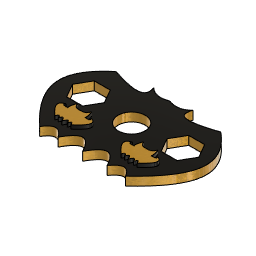
batman_fidget_spinner_darshan_nair (Autodesk Fusion 360 design; units mm, degrees)
Autodesk Fusion 360 part; units mm, degrees
sketch "Sketch1" plane through (0, 0, 0) normal (0, 0, 1) x (1, 0, 0)
  line L0 (0, 0) -> (0, 11)
  spline S0 degree 5 poles (0, 31) (0.3798, 30.869) (1.1341, 30.6235) (2.2502, 30.3047) (3.7068, 29.9801) (5.4716, 29.7535) (7.1751, 29.7226) (8.812, 29.9045) (10.3789, 30.3103) (11.8777, 30.9337) (13.3133, 31.7593) (14.4152, 32.5687) (15.217, 33.2543) (15.7408, 33.7457) (16, 34) knots 0 0 0 0 0 0 0.1 0.2 0.3 0.4 0.5 0.6 0.7 0.8 0.9 1 1 1 1 1 1
  spline S1 degree 5 poles (16, 34) (15.7635, 33.3498) (15.3667, 32.1059) (15.0006, 30.4093) (14.9782, 28.4915) (15.7664, 26.6977) (17.4106, 25.5367) (19.9066, 25.0054) (23.1867, 25.0538) (27.1658, 25.6189) (31.7601, 26.6389) (35.8754, 27.78) (39.1911, 28.8054) (41.5017, 29.563) (42.6821, 29.9604) knots 0 0 0 0 0 0 0.1 0.2 0.3 0.4 0.5 0.6 0.7 0.8 0.9 1 1 1 1 1 1
  spline S2 degree 5 poles (42.6821, 29.9604) (44.1584, 28.7477) (46.9634, 26.3054) (50.7286, 22.5913) (54.8497, 17.5364) (58.4053, 11.0351) (60.241, 4.3371) (60.2452, -2.5706) (58.4098, -9.6887) (54.8568, -17.0034) (49.7384, -24.4973) (44.5047, -30.6226) (39.9812, -35.2851) (36.704, -38.4234) (35, -40) knots 0 0 0 0 0 0 0.1 0.2 0.3 0.4 0.5 0.6 0.7 0.8 0.9 1 1 1 1 1 1
  spline S3 degree 5 poles (35, -40) (34.7252, -39.5521) (34.1734, -38.6959) (33.3391, -37.5297) (32.2132, -36.2152) (30.7816, -34.9998) (29.3239, -34.2492) (27.8379, -33.9997) (26.3228, -34.2679) (24.7799, -35.0299) (23.2114, -36.247) (21.9378, -37.5541) (20.9727, -38.7099) (20.3249, -39.5572) (20, -40) knots 0 0 0 0 0 0 0.1 0.2 0.3 0.4 0.5 0.6 0.7 0.8 0.9 1 1 1 1 1 1
  spline S4 degree 5 poles (20, -40) (19.6, -39.2415) (18.8, -37.7908) (17.6, -35.8134) (16, -33.581) (14, -31.5094) (12, -30.2211) (10, -29.7801) (8, -30.2211) (6, -31.5094) (4, -33.581) (2.4, -35.8134) (1.2, -37.7908) (0.4, -39.2415) (0, -40) knots 0 0 0 0 0 0 0.1 0.2 0.3 0.4 0.5 0.6 0.7 0.8 0.9 1 1 1 1 1 1
  spline S5 degree 5 poles (0, 31) (-0.3798, 30.869) (-1.1341, 30.6235) (-2.2502, 30.3047) (-3.7068, 29.9801) (-5.4716, 29.7535) (-7.1751, 29.7226) (-8.812, 29.9045) (-10.3789, 30.3103) (-11.8777, 30.9337) (-13.3133, 31.7593) (-14.4152, 32.5687) (-15.217, 33.2543) (-15.7408, 33.7457) (-16, 34) knots 0 0 0 0 0 0 0.1 0.2 0.3 0.4 0.5 0.6 0.7 0.8 0.9 1 1 1 1 1 1
  line L1 (-1.8866, 31.6508) -> (1.8866, 30.3492)
  line L2 (14.6318, 32.6578) -> (17.3682, 35.3422)
  line L3 (1.8866, 31.6508) -> (-1.8866, 30.3492)
  line L4 (-14.6318, 32.6578) -> (-17.3682, 35.3422)
  spline S6 degree 5 poles (-16, 34) (-15.7635, 33.3498) (-15.3667, 32.1059) (-15.0006, 30.4093) (-14.9782, 28.4915) (-15.7664, 26.6977) (-17.4106, 25.5367) (-19.9066, 25.0054) (-23.1867, 25.0538) (-27.1658, 25.6189) (-31.7601, 26.6389) (-35.8754, 27.78) (-39.1911, 28.8054) (-41.5017, 29.563) (-42.6821, 29.9604) knots 0 0 0 0 0 0 0.1 0.2 0.3 0.4 0.5 0.6 0.7 0.8 0.9 1 1 1 1 1 1
  line L5 (17.5567, 38.2791) -> (14.4433, 29.7209)
  line L6 (38.3421, 28.4994) -> (47.0222, 31.4213)
  line L7 (-17.5567, 38.2791) -> (-14.4433, 29.7209)
  line L8 (-38.3421, 28.4994) -> (-47.0222, 31.4213)
  spline S7 degree 5 poles (-42.6821, 29.9604) (-44.1584, 28.7477) (-46.9634, 26.3054) (-50.7286, 22.5913) (-54.8497, 17.5364) (-58.4053, 11.0351) (-60.241, 4.3371) (-60.2452, -2.5706) (-58.4098, -9.6887) (-54.8568, -17.0034) (-49.7384, -24.4973) (-44.5047, -30.6226) (-39.9812, -35.2851) (-36.704, -38.4234) (-35, -40) knots 0 0 0 0 0 0 0.1 0.2 0.3 0.4 0.5 0.6 0.7 0.8 0.9 1 1 1 1 1 1
  line L9 (34.9577, 36.3058) -> (50.4066, 23.6149)
  line L10 (42.7125, -32.864) -> (27.2875, -47.136)
  line L11 (-34.9577, 36.3058) -> (-50.4066, 23.6149)
  line L12 (-42.7125, -32.864) -> (-27.2875, -47.136)
  spline S8 degree 5 poles (-35, -40) (-34.7252, -39.5521) (-34.1734, -38.6959) (-33.3391, -37.5297) (-32.2132, -36.2152) (-30.7816, -34.9998) (-29.3239, -34.2492) (-27.8379, -33.9997) (-26.3228, -34.2679) (-24.7799, -35.0299) (-23.2114, -36.247) (-21.9378, -37.5541) (-20.9727, -38.7099) (-20.3249, -39.5572) (-20, -40) knots 0 0 0 0 0 0 0.1 0.2 0.3 0.4 0.5 0.6 0.7 0.8 0.9 1 1 1 1 1 1
  line L13 (36.1955, -41.9484) -> (33.8045, -38.0516)
  line L14 (21.3607, -38.1457) -> (18.6393, -41.8543)
  line L15 (-36.1955, -41.9484) -> (-33.8045, -38.0516)
  line L16 (-21.3607, -38.1457) -> (-18.6393, -41.8543)
  spline S9 degree 5 poles (-20, -40) (-19.6, -39.2415) (-18.8, -37.7908) (-17.6, -35.8134) (-16, -33.581) (-14, -31.5094) (-12, -30.2211) (-10, -29.7801) (-8, -30.2211) (-6, -31.5094) (-4, -33.581) (-2.4, -35.8134) (-1.2, -37.7908) (-0.4, -39.2415) (0, -40) knots 0 0 0 0 0 0 0.1 0.2 0.3 0.4 0.5 0.6 0.7 0.8 0.9 1 1 1 1 1 1
  line L17 (21.5767, -42.9909) -> (18.4233, -37.0091)
  line L18 (1.5794, -37.0105) -> (-1.5794, -42.9895)
  line L19 (-21.5767, -42.9909) -> (-18.4233, -37.0091)
  line L20 (-1.5794, -37.0105) -> (1.5794, -42.9895)
  circle A0 centre (0, 0) radius 11.05
  spline S10 degree 5 poles (-27, -15) (-26.7311, -15.0239) (-26.2109, -15.056) (-25.4835, -15.0575) (-24.6198, -14.9657) (-23.7179, -14.6962) (-22.9921, -14.2817) (-22.4353, -13.7442) (-22.0319, -13.1243) (-21.7558, -12.4856) (-21.5648, -11.9235) (-21.41, -11.5448) (-21.2469, -11.4404) (-21.0459, -11.6596) (-20.8038, -12.1839) (-20.5351, -12.9481) (-20.2662, -13.8594) (-20.0277, -14.8166) (-19.8481, -15.7276) (-19.7461, -16.5309) (-19.7315, -17.1925) (-19.793, -17.5959) (-19.8805, -17.826) (-19.9571, -17.9474) (-20, -18) knots 0 0 0 0 0 0 0.05 0.1 0.15 0.2 0.25 0.3 0.35 0.4 0.45 0.5 0.55 0.6 0.65 0.7 0.75 0.8 0.85 0.9 0.95 1 1 1 1 1 1
  spline S11 degree 5 poles (-20, -18) (-19.8028, -18.0252) (-19.4192, -18.0705) (-18.8763, -18.1231) (-18.2187, -18.1622) (-17.5153, -18.1555) (-16.9428, -18.0872) (-16.5158, -17.9507) (-16.247, -17.7399) (-16.1405, -17.4529) (-16.1886, -17.0932) (-16.3429, -16.7512) (-16.5199, -16.4659) (-16.6648, -16.263) (-16.7439, -16.1585) knots 0 0 0 0 0 0 0.1 0.2 0.3 0.4 0.5 0.6 0.7 0.8 0.9 1 1 1 1 1 1
  spline S12 degree 5 poles (-16.7439, -16.1585) (-16.3983, -16.2667) (-15.7473, -16.4977) (-14.8916, -16.8873) (-13.9963, -17.4948) (-13.31, -18.4093) (-13.0827, -19.4881) (-13.3268, -20.7358) (-14.0178, -22.1436) (-15.1134, -23.6964) (-16.5698, -25.3783) (-17.9943, -26.8168) (-19.1984, -27.9443) (-20.0604, -28.7171) (-20.5062, -29.1089) knots 0 0 0 0 0 0 0.1 0.2 0.3 0.4 0.5 0.6 0.7 0.8 0.9 1 1 1 1 1 1
  spline S13 degree 5 poles (-20.5062, -29.1089) (-20.569, -28.9494) (-20.694, -28.6442) (-20.8796, -28.2281) (-21.123, -27.7579) (-21.4202, -27.3209) (-21.7096, -27.0482) (-21.9906, -26.9535) (-22.2628, -27.0449) (-22.5265, -27.3155) (-22.7823, -27.7523) (-22.9813, -28.2238) (-23.1274, -28.6417) (-23.2235, -28.9485) (-23.2712, -29.1089) knots 0 0 0 0 0 0 0.1 0.2 0.3 0.4 0.5 0.6 0.7 0.8 0.9 1 1 1 1 1 1
  spline S14 degree 5 poles (-23.2712, -29.1089) (-23.3428, -28.931) (-23.4861, -28.5927) (-23.7019, -28.1378) (-23.9913, -27.6381) (-24.3561, -27.2031) (-24.724, -26.9733) (-25.0953, -26.963) (-25.4701, -27.176) (-25.8482, -27.5991) (-26.2293, -28.2145) (-26.5363, -28.8471) (-26.7677, -29.3953) (-26.9225, -29.7931) (-27, -30) knots 0 0 0 0 0 0 0.1 0.2 0.3 0.4 0.5 0.6 0.7 0.8 0.9 1 1 1 1 1 1
  spline S15 degree 5 poles (-27, -15) (-27.2689, -15.0239) (-27.7891, -15.056) (-28.5165, -15.0575) (-29.3802, -14.9657) (-30.2821, -14.6962) (-31.0079, -14.2817) (-31.5647, -13.7442) (-31.9681, -13.1243) (-32.2442, -12.4856) (-32.4352, -11.9235) (-32.59, -11.5448) (-32.7531, -11.4404) (-32.9541, -11.6596) (-33.1962, -12.1839) (-33.4649, -12.9481) (-33.7338, -13.8594) (-33.9723, -14.8166) (-34.1519, -15.7276) (-34.2539, -16.5309) (-34.2685, -17.1925) (-34.207, -17.5959) (-34.1195, -17.826) (-34.0429, -17.9474) (-34, -18) knots 0 0 0 0 0 0 0.05 0.1 0.15 0.2 0.25 0.3 0.35 0.4 0.45 0.5 0.55 0.6 0.65 0.7 0.75 0.8 0.85 0.9 0.95 1 1 1 1 1 1
  line L21 (-28.8323, -14.8373) -> (-25.1677, -15.1627)
  line L22 (-19.6155, -17.5281) -> (-20.3845, -18.4719)
  line L23 (-25.1677, -14.8373) -> (-28.8323, -15.1627)
  line L24 (-34.3845, -17.5281) -> (-33.6155, -18.4719)
  spline S16 degree 5 poles (-34, -18) (-34.1972, -18.0252) (-34.5808, -18.0705) (-35.1237, -18.1231) (-35.7813, -18.1622) (-36.4847, -18.1555) (-37.0572, -18.0872) (-37.4842, -17.9507) (-37.753, -17.7399) (-37.8595, -17.4529) (-37.8114, -17.0932) (-37.6571, -16.7512) (-37.4801, -16.4659) (-37.3352, -16.263) (-37.2561, -16.1585) knots 0 0 0 0 0 0 0.1 0.2 0.3 0.4 0.5 0.6 0.7 0.8 0.9 1 1 1 1 1 1
  line L25 (-20.8315, -17.8938) -> (-19.1685, -18.1062)
  line L26 (-16.2099, -16.8641) -> (-17.2779, -15.4529)
  line L27 (-33.1685, -17.8938) -> (-34.8315, -18.1062)
  line L28 (-37.7901, -16.8641) -> (-36.7221, -15.4529)
  spline S17 degree 5 poles (-37.2561, -16.1585) (-37.6017, -16.2667) (-38.2527, -16.4977) (-39.1084, -16.8873) (-40.0037, -17.4948) (-40.69, -18.4093) (-40.9173, -19.4881) (-40.6732, -20.7358) (-39.9822, -22.1436) (-38.8866, -23.6964) (-37.4302, -25.3783) (-36.0057, -26.8168) (-34.8016, -27.9443) (-33.9396, -28.7171) (-33.4938, -29.1089) knots 0 0 0 0 0 0 0.1 0.2 0.3 0.4 0.5 0.6 0.7 0.8 0.9 1 1 1 1 1 1
  line L29 (-19.1333, -15.4101) -> (-14.3545, -16.9069)
  line L30 (-18.5622, -27.4007) -> (-22.4501, -30.8171)
  line L31 (-34.8667, -15.4101) -> (-39.6455, -16.9069)
  line L32 (-35.4378, -27.4007) -> (-31.5499, -30.8171)
  spline S18 degree 5 poles (-33.4938, -29.1089) (-33.431, -28.9494) (-33.306, -28.6442) (-33.1204, -28.2281) (-32.877, -27.7579) (-32.5798, -27.3209) (-32.2904, -27.0482) (-32.0094, -26.9535) (-31.7373, -27.0449) (-31.4735, -27.3155) (-31.2177, -27.7523) (-31.0188, -28.2238) (-30.8726, -28.6417) (-30.7765, -28.9485) (-30.7288, -29.1089) knots 0 0 0 0 0 0 0.1 0.2 0.3 0.4 0.5 0.6 0.7 0.8 0.9 1 1 1 1 1 1
  line L33 (-20.2556, -29.745) -> (-20.7568, -28.4728)
  line L34 (-23.0751, -28.4497) -> (-23.4673, -29.7681)
  line L35 (-33.7444, -29.745) -> (-33.2432, -28.4728)
  line L36 (-30.9249, -28.4497) -> (-30.5327, -29.7681)
  spline S19 degree 5 poles (-30.7288, -29.1089) (-30.6572, -28.931) (-30.5139, -28.5927) (-30.2981, -28.1378) (-30.0087, -27.6381) (-29.6439, -27.2031) (-29.276, -26.9733) (-28.9047, -26.963) (-28.5299, -27.176) (-28.1518, -27.5991) (-27.7707, -28.2145) (-27.4637, -28.8471) (-27.2323, -29.3953) (-27.0775, -29.7931) (-27, -30) knots 0 0 0 0 0 0 0.1 0.2 0.3 0.4 0.5 0.6 0.7 0.8 0.9 1 1 1 1 1 1
  line L37 (-22.8739, -30.0971) -> (-23.6686, -28.1206)
  line L38 (-26.6353, -29.0266) -> (-27.3647, -30.9734)
  line L39 (-31.1261, -30.0971) -> (-30.3314, -28.1206)
  line L40 (-27.3647, -29.0266) -> (-26.6353, -30.9734)
  spline S20 degree 5 poles (27, -15) (26.7311, -15.0239) (26.2109, -15.056) (25.4835, -15.0575) (24.6198, -14.9657) (23.7179, -14.6962) (22.9921, -14.2817) (22.4353, -13.7442) (22.0319, -13.1243) (21.7558, -12.4856) (21.5648, -11.9235) (21.41, -11.5448) (21.2469, -11.4404) (21.0459, -11.6596) (20.8038, -12.1839) (20.5351, -12.9481) (20.2662, -13.8594) (20.0277, -14.8166) (19.8481, -15.7276) (19.7461, -16.5309) (19.7315, -17.1925) (19.793, -17.5959) (19.8805, -17.826) (19.9571, -17.9474) (20, -18) knots 0 0 0 0 0 0 0.05 0.1 0.15 0.2 0.25 0.3 0.35 0.4 0.45 0.5 0.55 0.6 0.65 0.7 0.75 0.8 0.85 0.9 0.95 1 1 1 1 1 1
  line L41 (28.8323, -14.8373) -> (25.1677, -15.1627)
  line L42 (19.6155, -17.5281) -> (20.3845, -18.4719)
  spline S21 degree 5 poles (27, -15) (27.2689, -15.0239) (27.7891, -15.056) (28.5165, -15.0575) (29.3802, -14.9657) (30.2821, -14.6962) (31.0079, -14.2817) (31.5647, -13.7442) (31.9681, -13.1243) (32.2442, -12.4856) (32.4352, -11.9235) (32.59, -11.5448) (32.7531, -11.4404) (32.9541, -11.6596) (33.1962, -12.1839) (33.4649, -12.9481) (33.7338, -13.8594) (33.9723, -14.8166) (34.1519, -15.7276) (34.2539, -16.5309) (34.2685, -17.1925) (34.207, -17.5959) (34.1195, -17.826) (34.0429, -17.9474) (34, -18) knots 0 0 0 0 0 0 0.05 0.1 0.15 0.2 0.25 0.3 0.35 0.4 0.45 0.5 0.55 0.6 0.65 0.7 0.75 0.8 0.85 0.9 0.95 1 1 1 1 1 1
  line L43 (25.1677, -14.8373) -> (28.8323, -15.1627)
  line L44 (34.3845, -17.5281) -> (33.6155, -18.4719)
  spline S22 degree 5 poles (34, -18) (34.1972, -18.0252) (34.5808, -18.0705) (35.1237, -18.1231) (35.7813, -18.1622) (36.4847, -18.1555) (37.0572, -18.0872) (37.4842, -17.9507) (37.753, -17.7399) (37.8595, -17.4529) (37.8114, -17.0932) (37.6571, -16.7512) (37.4801, -16.4659) (37.3352, -16.263) (37.2561, -16.1585) knots 0 0 0 0 0 0 0.1 0.2 0.3 0.4 0.5 0.6 0.7 0.8 0.9 1 1 1 1 1 1
  line L45 (33.1685, -17.8938) -> (34.8315, -18.1062)
  line L46 (37.7901, -16.8641) -> (36.7221, -15.4529)
  spline S23 degree 5 poles (37.2561, -16.1585) (37.6017, -16.2667) (38.2527, -16.4977) (39.1084, -16.8873) (40.0037, -17.4948) (40.69, -18.4093) (40.9173, -19.4881) (40.6732, -20.7358) (39.9822, -22.1436) (38.8866, -23.6964) (37.4302, -25.3783) (36.0057, -26.8168) (34.8016, -27.9443) (33.9396, -28.7171) (33.4938, -29.1089) knots 0 0 0 0 0 0 0.1 0.2 0.3 0.4 0.5 0.6 0.7 0.8 0.9 1 1 1 1 1 1
  line L47 (34.8667, -15.4101) -> (39.6455, -16.9069)
  line L48 (35.4378, -27.4007) -> (31.5499, -30.8171)
  spline S24 degree 5 poles (33.4938, -29.1089) (33.431, -28.9494) (33.306, -28.6442) (33.1204, -28.2281) (32.877, -27.7579) (32.5798, -27.3209) (32.2904, -27.0482) (32.0094, -26.9535) (31.7373, -27.0449) (31.4735, -27.3155) (31.2177, -27.7523) (31.0188, -28.2238) (30.8726, -28.6417) (30.7765, -28.9485) (30.7288, -29.1089) knots 0 0 0 0 0 0 0.1 0.2 0.3 0.4 0.5 0.6 0.7 0.8 0.9 1 1 1 1 1 1
  line L49 (33.7444, -29.745) -> (33.2432, -28.4728)
  line L50 (30.9249, -28.4497) -> (30.5327, -29.7681)
  spline S25 degree 5 poles (30.7288, -29.1089) (30.6572, -28.931) (30.5139, -28.5927) (30.2981, -28.1378) (30.0087, -27.6381) (29.6439, -27.2031) (29.276, -26.9733) (28.9047, -26.963) (28.5299, -27.176) (28.1518, -27.5991) (27.7707, -28.2145) (27.4637, -28.8471) (27.2323, -29.3953) (27.0775, -29.7931) (27, -30) knots 0 0 0 0 0 0 0.1 0.2 0.3 0.4 0.5 0.6 0.7 0.8 0.9 1 1 1 1 1 1
  line L51 (31.1261, -30.0971) -> (30.3314, -28.1206)
  line L52 (27.3647, -29.0266) -> (26.6353, -30.9734)
  spline S26 degree 5 poles (23.2712, -29.1089) (23.3428, -28.931) (23.4861, -28.5927) (23.7019, -28.1378) (23.9913, -27.6381) (24.3561, -27.2031) (24.724, -26.9733) (25.0953, -26.963) (25.4701, -27.176) (25.8482, -27.5991) (26.2293, -28.2145) (26.5363, -28.8471) (26.7677, -29.3953) (26.9225, -29.7931) (27, -30) knots 0 0 0 0 0 0 0.1 0.2 0.3 0.4 0.5 0.6 0.7 0.8 0.9 1 1 1 1 1 1
  line L53 (22.8739, -30.0971) -> (23.6686, -28.1206)
  line L54 (26.6353, -29.0266) -> (27.3647, -30.9734)
  spline S27 degree 5 poles (20.5062, -29.1089) (20.569, -28.9494) (20.694, -28.6442) (20.8796, -28.2281) (21.123, -27.7579) (21.4202, -27.3209) (21.7096, -27.0482) (21.9906, -26.9535) (22.2628, -27.0449) (22.5265, -27.3155) (22.7823, -27.7523) (22.9813, -28.2238) (23.1274, -28.6417) (23.2235, -28.9485) (23.2712, -29.1089) knots 0 0 0 0 0 0 0.1 0.2 0.3 0.4 0.5 0.6 0.7 0.8 0.9 1 1 1 1 1 1
  line L55 (20.2556, -29.745) -> (20.7568, -28.4728)
  line L56 (23.0751, -28.4497) -> (23.4673, -29.7681)
  spline S28 degree 5 poles (16.7439, -16.1585) (16.3983, -16.2667) (15.7473, -16.4977) (14.8916, -16.8873) (13.9963, -17.4948) (13.31, -18.4093) (13.0827, -19.4881) (13.3268, -20.7358) (14.0178, -22.1436) (15.1134, -23.6964) (16.5698, -25.3783) (17.9943, -26.8168) (19.1984, -27.9443) (20.0604, -28.7171) (20.5062, -29.1089) knots 0 0 0 0 0 0 0.1 0.2 0.3 0.4 0.5 0.6 0.7 0.8 0.9 1 1 1 1 1 1
  line L57 (19.1333, -15.4101) -> (14.3545, -16.9069)
  line L58 (18.5622, -27.4007) -> (22.4501, -30.8171)
  spline S29 degree 5 poles (20, -18) (19.8028, -18.0252) (19.4192, -18.0705) (18.8763, -18.1231) (18.2187, -18.1622) (17.5153, -18.1555) (16.9428, -18.0872) (16.5158, -17.9507) (16.247, -17.7399) (16.1405, -17.4529) (16.1886, -17.0932) (16.3429, -16.7512) (16.5199, -16.4659) (16.6648, -16.263) (16.7439, -16.1585) knots 0 0 0 0 0 0 0.1 0.2 0.3 0.4 0.5 0.6 0.7 0.8 0.9 1 1 1 1 1 1
  line L59 (20.8315, -17.8938) -> (19.1685, -18.1062)
  line L60 (16.2099, -16.8641) -> (17.2779, -15.4529)
  line L61 (-45, -8) -> (-32, -8)
  line L62 (-32, -8) -> (-25.5, 3.2583)
  line L63 (-25.5, 3.2583) -> (-32, 14.5167)
  line L64 (-32, 14.5167) -> (-45, 14.5167)
  line L65 (-45, 14.5167) -> (-51.5, 3.2583)
  line L66 (-51.5, 3.2583) -> (-45, -8)
  line L67 (-45, -8) -> (-31, -8) construction
  line L68 (25.5, 3.2583) -> (32, 14.5167)
  line L69 (32, 14.5167) -> (45, 14.5167)
  line L70 (45, 14.5167) -> (51.5, 3.2583)
  line L71 (51.5, 3.2583) -> (45, -8)
  line L72 (32, -8) -> (25.5, 3.2583)
  line L73 (32, -8) -> (45, -8)
  point P0 (9, 30)
  point P1 (17, 26)
  point P2 (60, 0)
  point P3 (27.9578, -34.1298)
  point P4 (10, -30)
  point P5 (-9, 30)
  point P6 (-17, 26)
  point P7 (-60, 0)
  point P8 (-27.9578, -34.1298)
  point P9 (-10, -30)
  point P10 (-22, -13)
  point P11 (-21.2425, -11.5193)
  point P12 (-20, -15)
  point P13 (-16.3602, -17.8008)
  point P14 (-13.2009, -19.5768)
  point P15 (-22, -27)
  point P16 (-25, -27)
  point P17 (-32, -13)
  point P18 (-32.7575, -11.5193)
  point P19 (-34, -15)
  point P20 (-37.6398, -17.8008)
  point P21 (-40.7991, -19.5768)
  point P22 (-32, -27)
  point P23 (-29, -27)
  point P24 (22, -13)
  point P25 (21.2425, -11.5193)
  point P26 (20, -15)
  point P27 (32, -13)
  point P28 (32.7575, -11.5193)
  point P29 (34, -15)
  point P30 (37.6398, -17.8008)
  point P31 (40.7991, -19.5768)
  point P32 (32, -27)
  point P33 (29, -27)
  point P34 (25, -27)
  point P35 (22, -27)
  point P36 (13.2009, -19.5768)
  point P37 (16.3602, -17.8008)
  point P38 (-35, 0)
  point P39 (-38.5, 3.2583)
  dimension "d1" = 11
  dimension "d2" = 20
  dimension "d5" = 22.1
  dimension "d13" = 13
  dimension "d14" = 0
  constraint coincident L0.start A0.centre
  constraint vertical L0
  constraint midpoint S0.start L1
  constraint midpoint S0.end L2
  constraint midpoint S0.end L5
  constraint midpoint S1.end L6
  constraint midpoint S1.end L9
  constraint midpoint S2.end L10
  constraint midpoint S2.end L13
  constraint midpoint S3.end L14
  constraint midpoint S3.end L17
  constraint midpoint S4.end L18
  constraint midpoint S10.start L21
  constraint midpoint S10.end L22
  constraint midpoint S10.end L25
  constraint midpoint S11.end L26
  constraint midpoint S11.end L29
  constraint midpoint S12.end L30
  constraint midpoint S12.end L33
  constraint midpoint S13.end L34
  constraint midpoint S13.end L37
  constraint midpoint S14.end L38
  constraint horizontal L67
  measures "d1" distance of L0.start L0.end
  measures "d2" distance of L0.end S0.start
  measures "d5" diameter of A0
  measures "d13" distance of L61.start L61.end
  measures "d14" angle of L61 L67
extrude "Extrude4" add sketch "Sketch1" along normal blind 7
extrude "Extrude5" add sketch "Sketch1" along normal blind 10 contours S10 S11 S12 S13 S14 S15 S16 S17 S18 S19 | S20 S21 S22 S23 S24 S25 S26 S27 S28 S29
